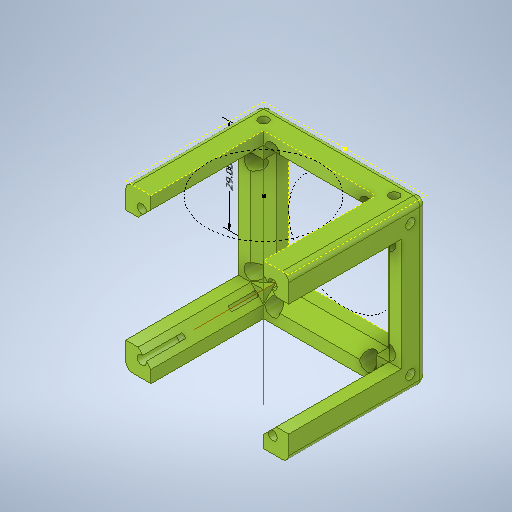
# Autodesk Inventor part: 10_Cube_1x1_v2
Saved by Autodesk Inventor 2025.1 (Build 291241000, 241)
## iProperties
Created: 2019-07-01
Part Number: 10_Cube_1x1_v2
Material: Generic
Document SubType Name: Modeling
Designer: diederichbenedict
Density: 1 g/cm^3
Appearance: IPHT_Grün
Author: diederichbenedict
Autodesk Inventor part; units mm, degrees
ref_plane "YZ Plane" through (0, 0, 0) normal (1, 0, 0) x (0, 1, 0)
ref_plane "XZ Plane" through (0, 0, 0) normal (0, 1, 0) x (-1, 0, 0)
ref_plane "XY Plane" through (0, 0, 0) normal (0, 0, 1) x (1, 0, 0)
sketch "Sketch1" plane through (0, 0, 0) normal (0, 0, 1) x (1, 0, 0)
  line L0 (-24.9, 24.9) -> (24.9, 24.9)
  line L1 (24.9, 24.9) -> (24.9, -24.9)
  line L2 (24.9, -24.9) -> (-24.9, -24.9)
  line L3 (-24.9, -24.9) -> (-24.9, 24.9)
  line L4 (-24.9, 24.9) -> (24.9, -24.9) construction
  line L5 (24.9, 24.9) -> (-24.9, -24.9) construction
  line L6 (17.2, 17.2) -> (-17.2, 17.2)
  line L7 (-17.2, 17.2) -> (-17.2, -17.2)
  line L8 (-17.2, -17.2) -> (17.2, -17.2)
  line L9 (17.2, -17.2) -> (17.2, 17.2)
  point P0 (0, 0)
  dimension "d0" = 49.8
  dimension "d1" = 49.8
  dimension "d2" = 7.7
  constraints: 20 end point, 4 parallel, 2 midpoint, 2 perpendicular, 1 horizontal, 3 other
  measures "d0" distance of L1.end L2.end
  measures "d1" distance of L0.end L1.end
  measures "d2" distance between parallel lines of L0 L6
extrude "Extrusion1" add sketch "Sketch1" along normal blind 7.7
sketch "Sketch2" plane through (0, 0, 7.7) normal (0, 0, 1) x (1, 0, 0)
  line L0 (17.2, 17.2) -> (17.2, -17.2) projected
  line L1 (17.2, -17.2) -> (-17.2, -17.2) projected
  line L2 (-17.2, -17.2) -> (-17.2, 17.2) projected
  line L3 (-17.2, 17.2) -> (17.2, 17.2) projected
  line L4 (24.9, 24.9) -> (-24.9, 24.9) projected
  line L5 (-24.9, 24.9) -> (-24.9, -24.9) projected
  line L6 (-24.9, -24.9) -> (24.9, -24.9) projected
  line L7 (24.9, -24.9) -> (24.9, 24.9) projected
  line L8 (17.2, -17.2) -> (24.9, -17.2)
  line L9 (24.9, -17.2) -> (24.9, -24.9)
  line L10 (24.9, -24.9) -> (17.2, -24.9)
  line L11 (17.2, -24.9) -> (17.2, -17.2)
  line L12 (17.2, 17.2) -> (-17.2, 17.2) projected
  line L13 (24.9, 24.9) -> (17.2, 24.9)
  line L14 (17.2, 24.9) -> (17.2, 17.2)
  line L15 (17.2, 17.2) -> (24.9, 17.2)
  line L16 (24.9, 17.2) -> (24.9, 24.9)
  line L17 (-24.9, -24.9) -> (-17.2, -24.9)
  line L18 (-17.2, -24.9) -> (-17.2, -17.2)
  line L19 (-17.2, -17.2) -> (-24.9, -17.2)
  line L20 (-24.9, -17.2) -> (-24.9, -24.9)
  line L21 (-24.9, 24.9) -> (-17.2, 24.9)
  line L22 (-17.2, 24.9) -> (-17.2, 17.2)
  line L23 (-17.2, 17.2) -> (-24.9, 17.2)
  line L24 (-24.9, 17.2) -> (-24.9, 24.9)
  point P0 (0, 0)
  constraints: 32 end point, 8 parallel, 4 horizontal, 4 perpendicular
extrude "Extrusion2" add sketch "Sketch2" along normal blind 34.4 contours L14 L4 L7 L15 | L8 L7 L6 L11 | L23 L5 L4 L22 | L18 L6 L5 L19
sketch "Sketch3" plane through (0, 0, 0) normal (0, 0, -1) x (-1, 0, 0)
  line L0 (24.9, -24.9) -> (24.9, 24.9) construction
  line L1 (24.9, 24.9) -> (-24.9, 24.9) construction
  line L2 (-24.9, -24.9) -> (24.9, -24.9) construction
  line L3 (-24.9, 24.9) -> (-24.9, -24.9) construction
  point P0 (20, 20)
  point P1 (20, -20)
  point P2 (-20, -20)
  point P3 (-20, 20)
  dimension "d_1" = 4.9
  dimension "d96" = 4.9
  dimension "d97" = 4.9
  dimension "d98" = 4.9
  dimension "d99" = 4.9
  dimension "d100" = 4.9
  dimension "d101" = 4.9
  dimension "d102" = 4.9
  measures "d_1" distance from line of L1 point (20, 20)
  measures "d96" distance from line of point (20, 20) L0
  measures "d97" distance from line of point (20, -20) L0
  measures "d98" distance from line of point (20, -20) L2
  measures "d99" distance from line of point (-20, -20) L2
  measures "d100" distance from line of point (-20, -20) L3
  measures "d101" distance from line of point (-20, 20) L3
  measures "d102" distance from line of point (-20, 20) L1
hole "Hole1" at (-20, 20, 0) at (-20, -20, 0) at (20, -20, 0) at (20, 20, 0) direction (0, 0, 1) diameter 2.8 depth 16 tip angle 118 counterbore diameter 5.5 counterbore depth 3.1
sketch "Sketch4" plane through (-24.9, 24.9, 0) normal (0, 1, 0) x (1, 0, 0)
  line L0 (0, 0) -> (49.8, 0) construction
  line L1 (0, 0) -> (0, -42.1) construction
  line L2 (7.7, -42.1) -> (0, -42.1) construction
  line L3 (7.7, -7.7) -> (7.7, -42.1) construction
  line L4 (42.1, -7.7) -> (7.7, -7.7) construction
  line L5 (42.1, -7.7) -> (42.1, -42.1) construction
  line L6 (49.8, -42.1) -> (42.1, -42.1) construction
  line L7 (49.8, 0) -> (49.8, -42.1) construction
  circle A0 centre (24.9, -24.9) radius 17.2 construction
  point P0 (24.9, 0)
  constraints: 3 tangent, 1 centre point
sketch "Sketch5" plane through (0, 0, 0) normal (0, 0, -1) x (-1, 0, 0)
  line L0 (-17.2, -17.2) -> (-17.2, 17.2) construction
  line L1 (-17.2, 17.2) -> (17.2, 17.2) construction
  line L2 (17.2, 17.2) -> (17.2, -17.2) construction
  line L3 (17.2, -17.2) -> (-17.2, -17.2) construction
  circle A0 centre (0, 0) radius 17.2 construction
  point P0 (0, 0)
  constraints: 3 tangent, 1 centre point
fillet "Fillet1" radius 2 8 edges at (24.9, 24.9, 21.05) (24.9, -24.9, 21.05) (-24.9, -24.9, 21.05) (-24.9, 24.9, 21.05) (-24.9, 0, 0) (0, -24.9, 0) (24.9, 0, 0) (0, 24.9, 0)
sketch "Sketch6" plane through (0, 0, 42.1) normal (0, 0, 1) x (1, 0, 0)
  arc A0 (-22.9, 24.9) -> (-24.9, 22.9) centre (-22.9, 22.9) ccw projected
  line L0 (-24.9, 22.9) -> (-24.9, 17.2) projected
  line L1 (-24.9, 17.2) -> (-17.2, 17.2) projected
  line L2 (-17.2, 17.2) -> (-17.2, 24.9) projected
  line L3 (-17.2, 24.9) -> (-22.9, 24.9) projected
  arc A1 (24.9, 22.9) -> (22.9, 24.9) centre (22.9, 22.9) ccw projected
  line L4 (22.9, 24.9) -> (17.2, 24.9) projected
  line L5 (17.2, 24.9) -> (17.2, 17.2) projected
  line L6 (17.2, 17.2) -> (24.9, 17.2) projected
  line L7 (24.9, 17.2) -> (24.9, 22.9) projected
  arc A2 (22.9, -24.9) -> (24.9, -22.9) centre (22.9, -22.9) ccw projected
  line L8 (24.9, -22.9) -> (24.9, -17.2) projected
  line L9 (24.9, -17.2) -> (17.2, -17.2) projected
  line L10 (17.2, -17.2) -> (17.2, -24.9) projected
  line L11 (17.2, -24.9) -> (22.9, -24.9) projected
  arc A3 (-24.9, -22.9) -> (-22.9, -24.9) centre (-22.9, -22.9) ccw projected
  line L12 (-22.9, -24.9) -> (-17.2, -24.9) projected
  line L13 (-17.2, -24.9) -> (-17.2, -17.2) projected
  line L14 (-17.2, -17.2) -> (-24.9, -17.2) projected
  line L15 (-24.9, -17.2) -> (-24.9, -22.9) projected
  line L16 (0, 38.1838) -> (54, 38.1838) construction
  line L17 (21.1252, 17.2) -> (17.2, 21.1252)
  line L18 (17.2, 24.9) -> (17.2, 17.2) projected
  line L19 (17.2, 21.1252) -> (17.2, 17.2)
  line L20 (17.2, 17.2) -> (21.1252, 17.2)
  line L21 (-17.2, 24.9) -> (-17.2, 17.2) projected
  line L22 (-17.2, 17.2) -> (-17.2, 21.1252)
  line L23 (-17.2, 21.1252) -> (-21.1252, 17.2)
  line L24 (-17.2, 21.1252) -> (-11.6489, 21.1252) construction
  line L25 (-17.2, -17.2) -> (-17.2, 17.2) projected
  line L26 (-21.1252, 17.2) -> (-17.2, 17.2)
  line L27 (-17.2, 17.2) -> (-21.1252, 17.2)
  line L28 (17.2, -17.2) -> (17.2, -24.9) projected
  line L29 (17.2, -17.2) -> (21.1252, -17.2)
  line L30 (24.9, -17.2) -> (17.2, -17.2) projected
  line L31 (21.1252, -17.2) -> (17.2, -21.1252)
  line L32 (17.2, -17.2) -> (17.2, -21.1252)
  line L33 (-17.2, -17.2) -> (-21.1252, -17.2)
  line L34 (-17.2, -17.2) -> (-17.2, -24.9) projected
  line L35 (-17.2, -17.2) -> (-17.2, -21.1252)
  line L36 (-21.1252, -17.2) -> (-17.2, -21.1252)
  line L37 (22.9, 22.9) -> (24.9, 22.9) construction
  line L38 (-22.9, -22.9) -> (22.9, 22.9) construction
  line L39 (-22.9, -22.9) -> (22.9, -22.9) construction
  line L40 (22.9, 22.9) -> (-22.9, 22.9) construction
  line L41 (22.9, -22.9) -> (-22.9, 22.9) construction
  dimension "d111" = 0
  dimension "d120" = 54.2
  dimension "d121" = 54.2
  constraints: 34 end point, 9 point on line, 3 collinear, 3 perpendicular, 2 horizontal, 1 equal length, 1 parallel, 1 vertical, 1 other
  measures "d111" vertical distance of L35.end L31.end
  measures "d120" distance between parallel lines of L31 L23
  measures "d121" distance between parallel lines of L36 L17
extrude "Extrusion3" cut sketch "Sketch6" against normal up to surface (34.4 mm away) contours L2 L1 L23 | L6 L5 L17 | L10 L9 L31 | L14 L13 L36
sketch "Sketch7" plane through (-24.9, 17.2, 7.7) normal (0, -1, 0) x (1, 0, 0)
  line L0 (42.1, 0) -> (50.1, 0) construction
  line L1 (42.1, -7.7) -> (42.1, 0) construction
  line L2 (7.7, -7.7) -> (7.7, 0) construction
  line L3 (-0.3, 0) -> (7.7, 0) construction
  line L4 (42.0475, 33.6419) -> (42.1, 0) construction
  line L5 (7.7, 0) -> (7.7521, 33.3764) construction
  line L6 (42.1, 0) -> (7.7, 0) construction
  circle A0 centre (24.9, 17.1732) radius 17.1732 construction
  line L7 (24.9, 55.4984) -> (-13.4252, 17.1732) construction
  line L8 (-13.4252, 17.1732) -> (24.9, -21.152) construction
  line L9 (24.9, -21.152) -> (63.2252, 17.1732) construction
  line L10 (63.2252, 17.1732) -> (24.9, 55.4984) construction
  line L11 (24.9, 55.4984) -> (24.9, -21.152) construction
  line L12 (-13.4252, 17.1732) -> (63.2252, 17.1732) construction
  line L13 (24.9, 55.4984) -> (79.1, 55.4984) construction
  line L14 (46.1838, 0) -> (42.1, 0)
  line L15 (46.1838, 0) -> (42.1, -3.952)
  line L16 (42.1, 0) -> (42.0475, 33.6419)
  line L17 (42.1, 0) -> (42.1, -3.952)
  line L18 (46.1838, 0) -> (42.1, 0)
  line L19 (42.1, 0) -> (46.1838, 0)
  line L20 (7.7, 0) -> (3.6162, 0)
  line L21 (3.6162, 0) -> (7.7, -3.952)
  line L22 (7.7, -3.952) -> (7.7, 0)
  line L23 (24.9, -36.4821) -> (24.9, 70.8284) projected
  point P0 (44.386, 0)
  point P1 (43.5978, 0)
  point P2 (24.9, 17.1732)
  dimension "d37" = 54.2
  dimension "d38" = 135
  dimension "d39" = 54.2
  constraints: 40 end point, 4 midpoint, 4 point on line, 3 collinear, 3 tangent, 2 horizontal, 2 parallel, 1 centre point, 1 equal length, 1 perpendicular, 1 vertical, 1 other
  measures "d37" distance of L7.start L7.end
  measures "d38" angle of L7 L13
  measures "d39" distance of L8.end L7.end
extrude "Extrusion4" cut sketch "Sketch7" along normal up to surface (34.4 mm away)
sketch "Sketch8" plane through (17.2, -24.9, 7.7) normal (-1, 0, 0) x (0, 0, 1)
  line L0 (-3.7838, 42.1) -> (0, 42.1) construction
  line L1 (-3.7838, 7.7) -> (0.3003, 7.7) construction
  line L2 (0.3003, 7.7) -> (0.3003, 3.6159) construction
  line L3 (-3.7838, 7.7) -> (0.3003, 3.6159)
  line L4 (0.3003, 3.6159) -> (0.3003, 7.7)
  line L5 (0.3003, 7.7) -> (-3.7838, 7.7)
  line L6 (-3.7838, 42.1) -> (0, 45.8838)
  line L7 (-3.7838, 42.1) -> (1.5673, 42.1) construction
  line L8 (0.3003, 7.7) -> (0, 42.1)
  line L9 (0, 45.8838) -> (0, 42.1)
  line L10 (0, 42.1) -> (-3.7838, 42.1)
  line L11 (-6, 2) -> (-6, 47.8)
  line L12 (55.3838, 24.9) -> (17.2, 63.0838) construction
  line L13 (17.2, 63.0838) -> (-20.9838, 24.9) construction
  line L14 (-20.9838, 24.9) -> (17.2, -13.2838) construction
  line L15 (17.2, -13.2838) -> (55.3838, 24.9) construction
  line L16 (55.3838, 24.9) -> (-20.9838, 24.9) construction
  line L17 (17.2, 63.0838) -> (17.2, -13.2838) construction
  line L18 (-36.2573, 24.9) -> (70.6573, 24.9) construction
  line L19 (17.2, -28.5573) -> (17.2, 78.3573) construction
  line L20 (0, 42.1) -> (0, 43.5346) construction
  line L21 (0, 7.7) -> (-3.952, 7.7) construction
  line L22 (-3.952, 42.1) -> (-3.952, 7.7) construction
  line L23 (0, 42.1) -> (-3.952, 42.1) construction
  line L24 (0, 7.7) -> (0, 42.1) construction
  point P0 (-2.4341, 8)
  point P1 (0, 5.414)
  point P2 (17.2, 24.9)
  point P3 (17.2, 24.9)
  point P4 (17.2, 24.9)
  dimension "d122" = 54
  dimension "d123" = 54
  constraints: 32 end point, 6 midpoint, 4 collinear, 3 horizontal, 2 parallel, 2 perpendicular, 2 vertical, 1 equal length, 1 point on line, 6 other
  measures "d122" distance of L12.start L12.end
  measures "d123" distance of L14.end L12.start
ref_plane "Work Plane1" through (-20.32, -18.034, 19.8181) normal (-1, 0, 0) x (0, 0, 1)
extrude "Extrusion5" cut sketch "Sketch8" along normal up to surface (34.4 mm away)
sketch "Sketch9" plane through (0, 0, 42.1) normal (0, 0, 1) x (1, 0, 0)
  arc A0 (19.6906, 18.6346) -> (18.6346, 19.6906) centre (20, 20) ccw projected
  arc A1 (18.6346, -19.6906) -> (19.6906, -18.6346) centre (20, -20) ccw projected
  arc A2 (-19.6906, -18.6346) -> (-18.6346, -19.6906) centre (-20, -20) ccw projected
  arc A3 (-18.6346, 19.6906) -> (-19.6906, 18.6346) centre (-20, 20) ccw projected
hole "Hole2" at (20, 20, 42.1) at (-20, 20, 42.1) at (20, -20, 42.1) at (-20, -20, 42.1) direction (0, 0, -1) diameter 2.8 depth 12 tip angle 118
sketch "Sketch11" plane through (24.9, -17.2, 7.7) normal (1, 0, 0) x (0, 0, -1)
  line L0 (-34.4, 40.1) -> (5.7, 40.1) construction
  line L1 (-34.4, 34.4) -> (-34.4, 40.1) construction
  line L2 (0, 34.4) -> (-34.4, 34.4) construction
  line L3 (0, 0) -> (0, 34.4) construction
  line L4 (0, 0) -> (-34.4, 0) construction
  line L5 (-34.4, -5.7) -> (-34.4, 0) construction
  line L6 (5.7, -5.7) -> (-34.4, -5.7) construction
  line L7 (5.7, 40.1) -> (5.7, -5.7) construction
  line L8 (-34.4, -7.7) -> (5.7, -7.7) construction
  line L9 (7.7, -5.7) -> (7.7, 40.1) construction
  line L10 (7.7, 42.1) -> (-34.4, 42.1) construction
  line L11 (-34.4, -2.8) -> (2.8, -2.8) construction
  line L12 (2.8, -2.8) -> (2.8, 37.2) construction
  line L13 (2.8, 37.2) -> (-34.4, 37.2) construction
  line L14 (-34.4, 37.2) -> (-34.4, -2.8) construction
  point P0 (3.1, -3.1)
  point P1 (3.1, 36.9)
  point P2 (8, 22.6681)
  point P3 (8, 61.1319)
  dimension "d88" = 4.9
  dimension "d89" = 4.9
  dimension "d90" = 4.9
  constraints: 8 end point, 2 parallel, 1 horizontal, 1 perpendicular, 1 point on line, 1 other
  measures "d88" distance from line of L11.end L8
  measures "d89" distance between parallel lines of L10 L13
hole "Hole4" at (24.9, 20, 4.9) at (24.9, -20, 4.9) direction (-1, 0, 0) diameter 2.9 depth 6.5 tip angle 118
sketch "Sketch12" plane through (-17.2, -24.9, 7.7) normal (0, -1, 0) x (1, 0, 0)
  line L0 (-7.7, 34.4) -> (-7.7, -5.7) construction
  line L1 (-5.7, -7.7) -> (40.1, -7.7) construction
  line L2 (42.1, -5.7) -> (42.1, 34.4) construction
  line L3 (-5.7, -7.7) -> (40.1, -7.7) construction
  point P0 (-2.3319, -8)
  point P1 (36.1319, -8)
  point P2 (-2.8, -2.8)
  point P3 (37.2, -2.8)
  point P4 (37.6681, -8)
  dimension "d91" = 4.9
  dimension "d92" = 4.9
  dimension "d93" = 4.9
  dimension "d94" = 4.9
  constraints: 2 other
  measures "d91" distance from line of point (-2.8, -2.8) L0
  measures "d94" distance from line of L2 point (37.2, -2.8)
hole "Hole5" at (-20, -24.9, 4.9) at (20, -24.9, 4.9) direction (0, 1, 0) diameter 2.9 depth 6.5 tip angle 118
sketch "Sketch13" plane through (-24.9, -17.2, 7.7) normal (-1, 0, 0) x (0, 0, 1)
  circle A0 centre (-2.8, 37.2) radius 1.45 projected
  circle A1 centre (-2.8, -2.8) radius 1.45 projected
  point P0 (-3.6423, -3.1)
  constraints: 1 other
hole "Hole6" at (-24.9, 20, 4.9) at (-24.9, -20, 4.9) direction (1, 0, 0) diameter 2.9 depth 6.5 tip angle 118
sketch "Sketch14" plane through (-17.2, 24.9, 7.7) normal (0, 1, 0) x (1, 0, 0)
  circle A0 centre (37.2, 2.8) radius 1.45 projected
  circle A1 centre (-2.8, 2.8) radius 1.45 projected
hole "Hole7" at (-20, 24.9, 4.9) at (20, 24.9, 4.9) direction (0, -1, 0) diameter 2.9 depth 6.5 tip angle 118
sketch "Sketch15" plane through (0, 0, 0) normal (0, 0, -1) x (-1, 0, 0)
  line L0 (-17.2, -17.2) -> (-17.2, 17.2) construction
  line L1 (-17.2, 17.2) -> (17.2, 17.2) construction
  line L2 (17.2, 17.2) -> (17.2, -17.2) construction
  line L3 (17.2, -17.2) -> (-17.2, -17.2) construction
  circle A0 centre (-20, 20) radius 2.75 construction
  circle A1 centre (20, -20) radius 2.75 construction
  circle A2 centre (20, 20) radius 2.75 construction
  circle A3 centre (-20, -20) radius 2.75 construction
  line L4 (-22.9, 22.9) -> (22.9, 22.9) construction
  line L5 (-22.9, -22.9) -> (-22.9, 22.9) construction
  line L6 (22.9, -22.9) -> (-22.9, -22.9) construction
  line L7 (22.9, 22.9) -> (22.9, -22.9) construction
  line L8 (17.2, 20.9838) -> (-17.2, 20.9838) construction
  point P0 (0, 0)
  point P1 (-20.8, -14.5)
  point P2 (-14.5, -20.8)
  point P3 (14.5, -20.8)
  point P4 (20.8, -14.5)
  point P5 (20.8, 14.5)
  point P6 (14.5, 20.8)
  point P7 (-14.5, 20.8)
  point P8 (-20.8, 14.5)
hole "Hole8" at (14.5, -20.8, 0) at (20.8, -14.5, 0) at (-14.5, -20.8, 0) at (-20.8, -14.5, 0) at (-20.8, 14.5, 0) at (-14.5, 20.8, 0) at (14.5, 20.8, 0) at (20.8, 14.5, 0) direction (0, 0, 1) diameter 4.7 end through all
equation "\"d1\" = d0"
equation "\"d96\" = d_1"
equation "\"d97\" = d_1"
equation "\"d98\" = d_1"
equation "\"d99\" = d_1"
equation "\"d100\" = d_1"
equation "\"d101\" = d_1"
equation "\"d102\" = d_1"
equation "\"d121\" = d120"
equation "\"d39\" = d37"
body "Solid1"
